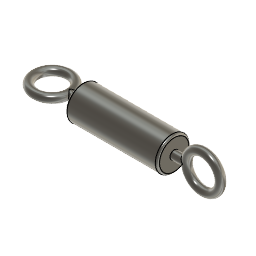
Assembled tag (Autodesk Fusion 360 archive; units mm, degrees)
design "GTR"
part number: 2026-04-07-14-43-03-079
Autodesk Fusion 360 part; units mm, degrees
torus "TorusPrimitive1" add centre line diameter 8 section diameter 2 placed x (1, 0, 0) y (0, 1, 0) z (0, 0, 1) at (0, 0, 0) makes body 1
ref_plane "WorkPlane1" through (4, 0, 0) normal (1, 0, 0) x (0, 1, 0)
cylinder "CylinderPrimitive1" add diameter 2 height 3 placed x (0, 0, -1) y (0, 1, 0) z (1, 0, 0) at (4, 0, 0) bodies 1
copy_body "CopyPasteBodies1" bodies 1 makes body 2
move_body "Move1" bodies 2 to x (-1, 0, 0) y (0, 1, 0) z (0, 0, -1) at (39, 0, -0.0001)
cylinder "CylinderPrimitive2" add diameter 8 height 22 placed x (0, 0, -1) y (0, 1, 0) z (1, 0, 0) at (7, 0, 0) bodies 1
move_body "Move2" bodies 2 to x (1, 0, 0) y (0, 0, 1) z (0, -1, 0) at (-3, -0.0001, -0.0001)
fillet "Fillet1" radius 0.5 1 edges at (7, 1.4465, 3.7293) on bodies 1
fillet "Fillet2" radius 0.5 1 edges at (29, -1.4465, 3.7293) on bodies 1

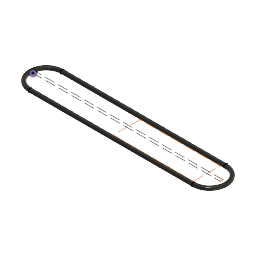
design "O-Ring"
part number: 2026-04-07-15-24-59-188
Autodesk Fusion 360 part; units mm, degrees
sketch "Sketch1" plane through (0, 0, 0) normal (0, 0, 1) x (1, 0, 0)
  line L0 (0, 0) -> (70, 0) construction
  line L1 (70, 0) -> (70, 1) construction
  line L2 (70, 1) -> (0, 1) construction
  line L3 (0, 1) -> (0, 0) construction
  line L4 (65, 5) -> (35, 5) construction
  line L5 (35, 5) -> (35, -5) construction
  line L6 (35, -5) -> (65, -5) construction
  line L7 (65, -5) -> (65, 5) construction
  dimension "d1" = 1
  constraint horizontal L0
  constraint vertical L1
  constraint horizontal L2
  constraint vertical L3
  constraint coincident L0.start L3.end
  constraint horizontal L4
  constraint vertical L5
  constraint horizontal L6
  constraint vertical L7
  measures "d1" distance of L0.start L2.end
sketch "Sketch2" plane through (0, 0, 0) normal (0, 0, 1) x (1, 0, 0)
sketch "Sketch9" plane through (0, 0, 0) normal (0, 0, 1) x (1, 0, 0)
  line L0 (5, -6) -> (66, -6)
  arc A0 (66, -6) -> (66, 6) centre (66, 0) ccw
  line L1 (66, 6) -> (5, 6)
  arc A1 (5, 6) -> (5, -6) centre (5, 0) ccw
  line L2 (5, 0) -> (66, 0) construction
  constraint tangent L0 A0
  constraint tangent A0 L1
  constraint parallel L0 L1
  constraint tangent L1 A1
  constraint tangent L0 A1
  constraint horizontal L2
pipe "Pipe3" add diameter 1.5 path "Sketch9" along L1 A1 L0 A0

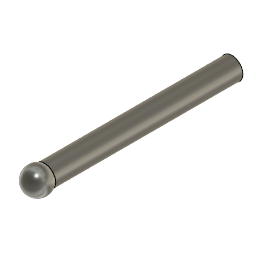
design "Release pin"
part number: 2025-10-28-15-51-31-568
Autodesk Fusion 360 part; units mm, degrees
sketch "Sketch1" plane through (0, 0, 0) normal (0, 1, 0) x (1, 0, 0)
  circle A0 centre (0, 0) radius 1.25
  dimension "d1" = 2.5
  constraint coincident A0.centre origin
  measures "d1" diameter of A0
extrude "Extrude1" add sketch "Sketch1" along normal blind 22
sphere "SpherePrimitive1" add diameter 3 placed x (1, 0, 0) y (0, 0, -1) z (0, 1, 0) at (0, 0, 0)

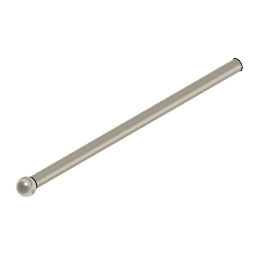
design "Main Pin"
part number: 2025-10-28-15-29-32-098
Autodesk Fusion 360 part; units mm, degrees
sketch "Sketch1" plane through (0, 0, 0) normal (0, 1, 0) x (1, 0, 0)
  circle A0 centre (1, -1) radius 1
  dimension "d1" = 2
  measures "d1" diameter of A0
extrude "Extrude1" add sketch "Sketch1" along normal blind 41 makes body 1
sphere "SpherePrimitive1" add diameter 3 placed x (1, 0, 0) y (0, 1, 0) z (0, 0, 1) at (1, -2, 0) separate body makes body 2
move_body "MoveFace1" bodies 2 to x (1, 0, 0) y (0, 1, 0) z (0, 0, 1) at (0, 1, 1) on bodies 2
combine "Combine1" operation add target body 2 tool bodies 1

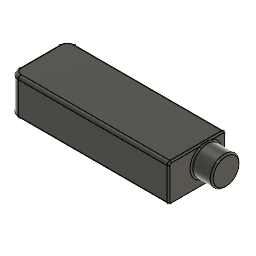
design "LittleLeo VDT3G"
part number: 2025-10-28-14-12-10-590
Autodesk Fusion 360 part; units mm, degrees
sketch "Sketch1" plane through (0, 0, 0) normal (0, 0, 1) x (1, 0, 0)
  line L0 (0, 0) -> (55, 0)
  line L1 (55, 0) -> (55, 20)
  line L2 (55, 20) -> (0, 20)
  line L3 (0, 20) -> (0, 0)
  dimension "d1" = 55
  dimension "d2" = 20
  constraint horizontal L0
  constraint vertical L1
  constraint horizontal L2
  constraint vertical L3
  constraint coincident L0.start L3.end
  measures "d1" distance of L0.start L0.end
  measures "d2" distance of L0.start L2.end
extrude "Extrude1" add sketch "Sketch1" along normal blind 13
sketch "Sketch2" plane through (55, 0, 0) normal (1, 0, 0) x (0, 1, 0)
  circle A0 centre (12.9791, 7.5121) radius 5
  dimension "d5" = 10
  measures "d5" diameter of A0
extrude "Extrude2" add sketch "Sketch2" along normal blind 7
fillet "Fillet1" radius 3 2 edges at (0, 20, 6.5) (0, 0, 6.5)
fillet "Fillet2" radius 1 5 edges at (29, 20, 13) (0.8787, 19.1213, 13) (0, 10, 13) (0.8787, 0.8787, 13) (29, 0, 13)
fillet "Fillet3" radius 1 5 edges at (29, 20, 0) (0.8787, 19.1213, 0) (0, 10, 0) (0.8787, 0.8787, 0) (29, 0, 0)
fillet "Fillet4" radius 0.5 1 faces at (55, 2.6783, 6.589)
fillet "Fillet5" radius 0.5 1 faces at (62, 14.4389, 8.7191)
